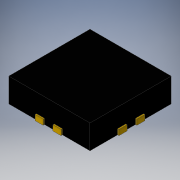
# Autodesk Inventor part: MC_DQ849
Saved by Autodesk Inventor 2016 (Build 200138000, 138)
## iProperties
Created: 2016-08-30
Part Number: MC_DQ849
Material: Generic
Document SubType Name: Modeling
Designer: jfixelle
Density: 1 g/cm^3
Appearance: Black
Author: jfixelle
Autodesk Inventor part; units mm, degrees
ref_plane "YZ Plane" through (0, 0, 0) normal (1, 0, 0) x (0, 1, 0)
ref_plane "XZ Plane" through (0, 0, 0) normal (0, 1, 0) x (-1, 0, 0)
ref_plane "XY Plane" through (0, 0, 0) normal (0, 0, 1) x (1, 0, 0)
sketch "Sketch1" plane through (0, 0, 0) normal (0, 1, 0) x (-1, 0, 0)
  line L0 (1.5, 1.5) -> (-1.5, 1.5)
  line L1 (-1.5, 1.5) -> (-1.5, -1.5)
  line L2 (-1.5, -1.5) -> (1.5, -1.5)
  line L3 (1.5, -1.5) -> (1.5, 1.5)
  point P0 (0, 0)
  dimension "d0" = 3
  dimension "d1" = 3
  dimension "d2" = 1.5
  dimension "d3" = 1.5
  constraints: 8 end point, 2 parallel, 1 horizontal, 1 perpendicular
  measures "d0" distance of L2.end L0.start
  measures "d1" distance of L1.end L2.end
  measures "d2" distance from line of L2 point (0, 0)
  measures "d3" distance from line of L3 point (0, 0)
extrude "Extrusion1" add sketch "Sketch1" along normal blind 0.89
sketch "Sketch2" plane through (0, 0, 0) normal (0, -1, 0) x (1, 0, 0)
  line L0 (1.55, 0.48) -> (1.14, 0.48)
  line L1 (1.14, 0.48) -> (1.14, 0.18)
  line L2 (1.14, 0.18) -> (1.55, 0.18)
  line L3 (1.55, 0.18) -> (1.55, 0.48)
  line L4 (1.5, 1.5) -> (1.5, -1.5) projected
  line L5 (-1.5, 1.5) -> (1.5, 1.5) projected
  point P0 (0, 0)
  dimension "d6" = 0.3
  dimension "d7" = 0.05
  dimension "d8" = 0.41
  dimension "d9" = 1.02
  constraints: 8 end point, 2 parallel, 1 horizontal, 1 perpendicular
  measures "d6" distance of L2.end L0.start
  measures "d7" distance between parallel lines of L4 L3
  measures "d8" distance of L1.end L2.end
  measures "d9" distance between parallel lines of L5 L0
extrude "Extrusion2" add sketch "Sketch2" against normal blind 0.2
mirror "Mirror1" about plane through (0, 0, 0) normal (0, 0, 1) of "Extrusion2"
pattern_circular "Circular Pattern1" count 4 over 360 about axis through (0, -10, 0) along (0, 1, 0) of "Extrusion2", "Mirror1"
body "Solid1"
